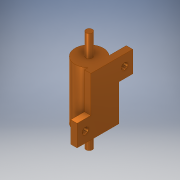
# Autodesk Inventor part: Power Resistor - HSA25
Saved by Autodesk Inventor 2017 (Build 210142000, 142)
## iProperties
Created: 2022-12-04
Part Number: Power Resistor - HSA25
Material: Gold
Document SubType Name: Modeling
Designer: Win240
Mass: 273.3 g
Surface Area: 53.5113 cm^2
Volume: 14.1606 cm^3
Density: 19.3 g/cm^3
Appearance: Metal 1600F Hot
Author: Win240
Autodesk Inventor part; units mm, degrees
ref_plane "YZ Plane" through (0, 0, 0) normal (1, 0, 0) x (0, 1, 0)
ref_plane "XZ Plane" through (0, 0, 0) normal (0, 1, 0) x (-1, 0, 0)
ref_plane "XY Plane" through (0, 0, 0) normal (0, 0, 1) x (1, 0, 0)
sketch "Sketch1" plane through (0, 0, 0) normal (0, 1, 0) x (-1, 0, 0)
  arc A0 (3.2, -5.3217) -> (15, 0) centre (7.9, 0) ccw
  line L0 (3.2, -5.3217) -> (3.2, -14)
  line L1 (3.2, -14) -> (0, -14)
  line L2 (0, -14) -> (0, 14)
  line L3 (0, 14) -> (3.2, 14)
  line L4 (3.2, 14) -> (3.2, 5.3217)
  arc A1 (15, 0) -> (3.2, 5.3217) centre (7.9, 0) ccw
  line L5 (7.9, 7.1) -> (7.9, -7.1) construction
  line L6 (3.2, 5.3217) -> (15, 0) construction
  line L7 (3.2, -5.3217) -> (15, 0) construction
  point P0 (0, 0)
  point P1 (0, 0)
  dimension "d0" = 3.2
  dimension "d1" = 28
  dimension "d5" = 14.2
  dimension "d6" = 15
  constraints: 16 end point, 6 point on circle, 4 vertical, 3 equal length, 2 centre point, 2 concentric, 2 horizontal, 2 line through centre, 1 coincident, 1 midpoint
  measures "d0" distance of L0.end L1.end
  measures "d1" distance of L1.end L2.end
  measures "d5" distance of L5.start L5.end
  measures "d6" distance from line of L6.end L2
extrude "Extrusion1" add sketch "Sketch1" along normal blind 29
sketch "Sketch2" plane through (0, 0, 14) normal (1, 0, 0) x (0, 0, -1)
  circle A0 centre (23.9, 23.65) radius 1.65
  circle A1 centre (4.1, 5.35) radius 1.65
  line L0 (23.9, 23.65) -> (23.9, 5.35) construction
  line L1 (23.9, 5.35) -> (4.1, 5.35) construction
  line L2 (28, 0) -> (28, 29) projected
  line L3 (0, 0) -> (0, 29) projected
  line L4 (23.9, 23.65) -> (28, 23.65) construction
  line L5 (23.9, 23.65) -> (28, 29) construction
  line L6 (0, 0) -> (4.1, 5.35) construction
  line L7 (4.1, 5.35) -> (0, 5.35) construction
  line L8 (28, 18.3) -> (21.1, 18.3)
  line L9 (21.1, 18.3) -> (21.1, 0)
  line L10 (21.1, 0) -> (28, 0)
  line L11 (0, 10.7) -> (6.9, 10.7)
  line L12 (6.9, 10.7) -> (6.9, 29)
  line L13 (6.9, 29) -> (0, 29)
  line L14 (28, 18.3) -> (23.9, 23.65) construction
  point P0 (14, 0)
  dimension "d9" = 19.8
  dimension "d10" = 18.3
  dimension "d11" = 3.3
  dimension "d12" = 2.8
  constraints: 26 end point, 7 horizontal, 5 equal length, 4 point on line, 3 vertical, 2 centre point, 1 equal radius
  measures "d9" distance of L0.end L1.end
  measures "d10" distance of L0.start L0.end
  measures "d11" diameter of A0
  measures "d12" distance from line of L0.start L9
extrude "Extrusion2" cut sketch "Sketch2" against normal up to surface (3.2 mm away)
sketch "Sketch3" plane through (0, 0, 0) normal (0, -1, 0) x (1, 0, 0)
  arc A0 (-3.2, 5.3217) -> (-3.2, -5.3217) centre (-7.9, 0) ccw projected
  circle A1 centre (-7.9, 0) radius 1.5875
  point P0 (0, 0)
  dimension "d15" = 3.175
  constraints: 1 centre point, 1 coincident
  measures "d15" diameter of A1
extrude "Extrusion3" add sketch "Sketch3" along normal blind 11
sketch "Sketch4" plane through (0, 29, 0) normal (0, 1, 0) x (1, 0, 0)
  arc A0 (-3.2, 5.3217) -> (-3.2, -5.3217) centre (-7.9, 0) ccw construction
  circle A1 centre (-7.9, 0) radius 1.5875
  point P0 (0, 0)
  dimension "d18" = 3.175
  constraints: 1 centre point, 1 coincident
  measures "d18" diameter of A1
extrude "Extrusion4" add sketch "Sketch4" along normal blind 11
body "Solid1"
